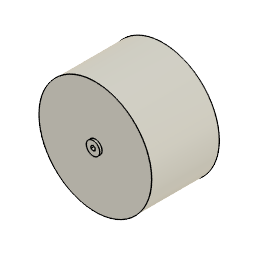
Rear Wheel (Autodesk Fusion 360 design; units mm, degrees)
Autodesk Fusion 360 part; units mm, degrees
sketch "スケッチ1" plane through (0, 0, 0) normal (0, 1, 0) x (1, 0, 0)
  circle A0 centre (0, 0) radius 25
  dimension "d1" = 50
  constraint coincident A0.centre origin
  measures "d1" diameter of A0
extrude "押し出し1" add sketch "スケッチ1" along normal blind 30
sketch "スケッチ2" plane through (0, 0, 0) normal (0, -1, 0) x (1, 0, 0)
  circle A0 centre (0, 0) radius 25
  circle A1 centre (0, 0) radius 3
  line L0 (0, 1.05) -> (-0.9093, 0.525)
  line L1 (-0.9093, 0.525) -> (-0.9093, -0.525)
  line L2 (-0.9093, -0.525) -> (0, -1.05)
  line L3 (0, -1.05) -> (0.9093, -0.525)
  line L4 (0.9093, -0.525) -> (0.9093, 0.525)
  line L5 (0.9093, 0.525) -> (0, 1.05)
  dimension "d4" = 6
  dimension "d5" = 2.1
  constraint coincident A0.centre A1.centre
  measures "d4" diameter of A1
  measures "d5" distance of L0.start L2.end
extrude "押し出し2" add sketch "スケッチ2" along normal blind 1 contours A1
extrude "押し出し3" cut 1 faces at (0, 0, 0.35) along direction (0, 1, 0) blind 4
